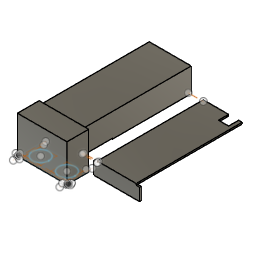
enclosure (Autodesk Fusion 360 design; units mm, degrees)
Autodesk Fusion 360 part; units mm, degrees
sketch "Sketch1" plane through (0, 0, 0) normal (0, 0, 1) x (1, 0, 0)
  line L0 (0, 0) -> (41.5, 0)
  line L1 (41.5, 0) -> (41.5, 105)
  line L2 (41.5, 105) -> (0, 105)
  line L3 (0, 105) -> (0, 0)
  dimension "d1" = 41.5
  dimension "d2" = 105
  constraint horizontal L0
  constraint vertical L1
  constraint horizontal L2
  constraint vertical L3
  constraint coincident L0.start L3.end
  measures "d1" distance of L0.start L0.end
  measures "d2" distance of L0.start L2.end
extrude "Extrude1" add sketch "Sketch1" along normal blind 23 makes body 1
sketch "Sketch2" plane through (0, 0, 0) normal (0, 0, -1) x (1, 0, 0)
  line L0 (0, 0) -> (0, -105)
  line L1 (0, -105) -> (41.5, -105)
  line L2 (41.5, -105) -> (41.5, 0)
  line L3 (41.5, 0) -> (0, 0)
  line L4 (0, -105) -> (41.5, -105)
  line L5 (41.5, -105) -> (41.5, -27)
  line L6 (41.5, -27) -> (0, -27)
  line L7 (0, -27) -> (0, -105)
  dimension "d5" = 78
  constraint horizontal L4
  constraint vertical L5
  constraint horizontal L6
  constraint vertical L7
  constraint coincident L0.end L1.start
  measures "d5" distance of L0.end L6.end
extrude "Extrude2" add sketch "Sketch2" along normal blind 0.75 contours L0 L1 L2 L4 L5 L6 L7 bodies 1
sketch "Sketch3" plane through (0, 0, 0) normal (0, 1, 0) x (1, 0, 0)
  line L0 (-4, 13.7485) -> (45, 13.7485)
  line L1 (45, 13.7485) -> (45, -20.0015)
  line L2 (45, -20.0015) -> (-4, -20.0015)
  line L3 (-4, -20.0015) -> (-4, 13.7485)
  line L4 (20.5, -20.0015) -> (20.5, 1) construction
  dimension "d8" = 49
  dimension "d9" = 33.75
  constraint midpoint L2 L4.start
  constraint perpendicular L2 L4
  constraint symmetric L1 L3 L4
  measures "d8" distance of L0.start L0.end
  measures "d9" distance of L0.start L2.end
extrude "Extrude3" add sketch "Sketch3" against normal blind 21.5 bodies 1
move_face "OffsetFaces1" offset 3 1 faces at (13.6667, -14.3333, 20.0015) on bodies 1
shell "Shell1" thickness 1.5 removed faces 2 at (13.8333, 18, 0) at (13.8333, 79, -0.75) on bodies 1
sketch "Sketch4" plane through (0, 0, -0.75) normal (0, 0, -1) x (1, 0, 0)
  line L0 (40, -103.5) -> (1.5, -103.5)
  line L1 (1.5, -103.5) -> (1.5, -28.5)
  line L2 (1.5, -28.5) -> (40, -28.5)
  line L3 (40, -28.5) -> (40, -103.5)
  line L4 (0, -27) -> (0, -105)
  line L5 (0, -105) -> (41.5, -105)
  line L6 (41.5, -105) -> (41.5, -27)
  line L7 (41.5, -27) -> (0, -27)
surface "Extrude4" add extruded along (0, 1, 0) between 0 and -1.5 1 faces at (27.1667, 28.5, -0.25) separate body on bodies 1 makes body 2
extrude "Extrude5" cut 1 faces at (27.1667, 28, -0.75) along direction (0, 0, 1) blind 1 on bodies 2 bodies 1 2
sketch "Sketch7" plane through (0, 0, 0) normal (0, 1, 0) x (-1, 0, 0)
  line L0 (4, 23.0015) -> (-45, 23.0015)
  line L1 (-45, 23.0015) -> (-45, -13.7485)
  line L2 (-45, -13.7485) -> (4, -13.7485)
  line L3 (4, -13.7485) -> (4, 23.0015)
  line L4 (0, 23) -> (0, 0)
  line L5 (0, 0) -> (-1.5, 0)
  line L6 (-1.5, 0) -> (-40, 0)
  line L7 (-40, 0) -> (-41.5, 0)
  line L8 (-41.5, 0) -> (-41.5, 23)
  line L9 (-41.5, 23) -> (0, 23)
  line L10 (4, -13.7485) -> (2.5, -13.7485) construction
  line L11 (2.5, -13.7485) -> (2.5, -12.2485) construction
  line L12 (-45, -13.7485) -> (-43.5, -13.7485) construction
  line L13 (-43.5, -13.7485) -> (-43.5, -12.2485) construction
  line L14 (4, 0) -> (-45, 0) construction
  dimension "d25" = 1.5
  dimension "d26" = 1.5
  dimension "d27" = 1.5
  dimension "d28" = 1.5
  constraint coincident L2.end L3.start
  constraint perpendicular L3 L10
  constraint perpendicular L10 L11
  constraint coincident L1.end L2.start
  constraint perpendicular L1 L12
  constraint perpendicular L12 L13
  constraint coincident L3 L14.start
  constraint perpendicular L4 L14
  measures "d25" distance of L2.end L10.end
  measures "d26" distance of L10.end L11.end
  measures "d27" distance of L1.end L12.end
  measures "d28" distance of L12.end L13.end
sketch "Sketch13" plane through (0, 0, 0) normal (0, 1, 0) x (-1, 0, 0)
  line L0 (2.5, -12.25) -> (-43.5, -12.25)
  line L1 (-43.5, -12.25) -> (-43.5, 0)
  line L2 (-43.5, 0) -> (2.5, 0)
  line L3 (2.5, 0) -> (2.5, -12.25)
  dimension "d29" = 46
  constraint horizontal L0
  constraint vertical L1
  constraint horizontal L2
  constraint vertical L3
  measures "d29" distance of L0.start L0.end
extrude "Extrude6" cut sketch "Sketch13" against normal blind 2 bodies 1
sketch "Sketch16" plane through (0, 0, -13.7485) normal (0, 0, -1) x (1, 0, 0)
  line L0 (-4, 0) -> (45, 0)
  line L1 (45, 0) -> (45, 21.5)
  line L2 (45, 21.5) -> (-4, 21.5)
  line L3 (-4, 21.5) -> (-4, 0)
  line L4 (-4, 21.5) -> (-2.5, 21.5) construction
  line L5 (45, 21.5) -> (43.5, 21.5) construction
  line L6 (-2.5, 27.1205) -> (-2.5, -5) construction
  line L7 (43.5, 27.0831) -> (43.5, -5) construction
  line L8 (-4, 21.5) -> (-4, 20) construction
  line L9 (45, 21.5) -> (45, 20) construction
  line L10 (-7, 20) -> (47, 20) construction
  line L11 (-2.5, 20) -> (-2.5, 18) construction
  line L12 (-5, 18) -> (46, 18) construction
  line L13 (-2.5, 18) -> (-0.5, 18) construction
  line L14 (-0.5, 22.9727) -> (-0.5, -1) construction
  line L15 (-0.5, 18) -> (15.5, 18) construction
  line L16 (15.5, 18) -> (15.5, 2) construction
  line L17 (15.5, 2) -> (-0.5, 2) construction
  line L18 (-0.5, 2) -> (-0.5, 18) construction
  line L19 (43.5, 20) -> (41.5, 20) construction
  line L20 (41.5, 22.2886) -> (41.5, -1) construction
  line L21 (41.5, 18) -> (25.5, 18) construction
  line L22 (25.5, 18) -> (25.5, 2) construction
  line L23 (25.5, 2) -> (41.5, 2) construction
  line L24 (41.5, 2) -> (41.5, 18) construction
  circle A0 centre (7.5, 10) radius 8
  circle A1 centre (33.5, 10) radius 8
  dimension "d35" = 1.5
  dimension "d36" = 1.5
  dimension "d37" = 2
  dimension "d38" = 16
  dimension "d39" = 16
  dimension "d40" = 2
  dimension "d41" = 16
  dimension "d42" = 16
  dimension "d43" = 8
  dimension "d44" = 8
  constraint coincident L2.end L3.start
  constraint perpendicular L3 L4
  constraint coincident L1.end L2.start
  constraint perpendicular L1 L5
  constraint perpendicular L2 L6
  constraint perpendicular L0 L7
  constraint coincident L3 L8.end
  constraint perpendicular L4 L8
  constraint coincident L1 L9.end
  constraint perpendicular L5 L9
  constraint perpendicular L8 L10
  constraint coincident L10 L11.start
  constraint coincident L6 L11.start
  constraint coincident L6 L11.end
  constraint perpendicular L10 L11
  constraint perpendicular L1 L12
  constraint perpendicular L11 L13
  constraint perpendicular L0 L14
  constraint horizontal L15
  constraint vertical L16
  constraint horizontal L17
  constraint vertical L18
  constraint coincident L10 L19.start
  constraint coincident L7 L19.start
  constraint perpendicular L7 L19
  constraint perpendicular L0 L20
  constraint horizontal L21
  constraint vertical L22
  constraint horizontal L23
  constraint vertical L24
  constraint coincident L20 L21.start
  constraint coincident L12 L21.start
  constraint tangent L17 A0
  constraint tangent L18 A0
  constraint tangent L23 A1
  constraint tangent L22 A1
  measures "d35" distance of L2.end L4.end
  measures "d36" distance of L1.end L5.end
  measures "d37" distance of L11.end L13.end
  measures "d38" distance of L13.end L15.end
  measures "d39" distance of L13.end L17.end
  measures "d40" distance of L19.start L19.end
  measures "d41" distance of L21.start L21.end
  measures "d42" distance of L21.start L23.end
  measures "d43" radius of A0
  measures "d44" radius of A1
extrude "Extrude7" add sketch "Sketch16" against normal blind 2 contours A1 bodies 1
extrude "Extrude8" cut sketch "Sketch16" against normal blind 2 contours A1 bodies 1
extrude "Extrude9" cut sketch "Sketch16" against normal blind 2 contours A0 bodies 1
sketch "Sketch17" plane through (0, 105, 0) normal (0, 1, 0) x (-1, 0, 0)
  line L0 (0, -0.75) -> (0, 23)
  line L1 (0, 23) -> (-41.5, 23)
  line L2 (-41.5, 23) -> (-41.5, -0.75)
  line L3 (-41.5, -0.75) -> (0, -0.75)
  line L4 (-41.5, -0.75) -> (-36.5, -0.75) construction
  line L5 (-36.5, -0.75) -> (-26.5, -0.75)
  line L6 (-26.5, -0.75) -> (-26.5, 4.25)
  line L7 (-26.5, 4.25) -> (-36.5, 4.25)
  line L8 (-36.5, 4.25) -> (-36.5, -0.75)
  dimension "d51" = 5
  dimension "d52" = 10
  dimension "d53" = 5
  constraint coincident L2.end L3.start
  constraint perpendicular L2 L4
  constraint horizontal L5
  constraint vertical L6
  constraint horizontal L7
  constraint vertical L8
  measures "d51" distance of L2.end L4.end
  measures "d52" distance of L4.end L5.end
  measures "d53" distance of L4.end L7.end
extrude "Extrude10" cut sketch "Sketch17" against normal blind 5 contours L3 L5 L6 L7 L8 bodies 1
sketch "Sketch18" plane through (0, 0, 0) normal (0, 0, 1) x (1, 0, 0)
  line L0 (50, 115) -> (88.6, 115)
  line L1 (88.6, 115) -> (88.6, 10)
  line L2 (88.6, 10) -> (50, 10)
  line L3 (50, 10) -> (50, 115)
  dimension "d56" = 38.6
  dimension "d57" = 105
  constraint horizontal L0
  constraint vertical L1
  constraint horizontal L2
  constraint vertical L3
  measures "d56" distance of L0.start L0.end
  measures "d57" distance of L0.start L2.end
extrude "Extrude11" add sketch "Sketch18" against normal blind 1.5 separate body makes body 3
delete_body "RemoveBody1" bodies 2
delete_body "RemoveBody2" bodies 3
sketch "Sketch19" plane through (0, 0, 0) normal (0, 0, 1) x (1, 0, 0)
sketch "Sketch20" plane through (0, 0, 0) normal (0, 0, 1) x (1, 0, 0)
  line L0 (40, 103.5) -> (55, 103.5) construction
  line L1 (40, 0) -> (55, 0) construction
  line L2 (40, -1.5) -> (55, -1.5) construction
  constraint horizontal L0
  constraint horizontal L1
  constraint parallel L1 L2
sketch "Sketch21" plane through (0, 0, 0) normal (0, 0, 1) x (1, 0, 0)
  line L0 (55, 103.5) -> (93.5, 103.5)
  line L1 (93.5, 103.5) -> (93.5, 0)
  line L2 (93.5, 0) -> (55, 0)
  line L3 (55, 0) -> (55, 103.5)
  line L4 (55, 0) -> (51.5, 0) construction
  line L5 (93.5, 0) -> (97, 0) construction
  dimension "d60" = 38.5
  dimension "d61" = 103.5
  dimension "d62" = 3.5
  constraint horizontal L0
  constraint vertical L1
  constraint horizontal L2
  constraint vertical L3
  constraint perpendicular L3 L4
  constraint perpendicular L1 L5
  measures "d60" distance of L0.start L0.end
  measures "d61" distance of L0.start L2.end
  measures "d62" distance of L2.end L4.end
sketch "Sketch24" plane through (0, 0, 0) normal (0, 1, 0) x (1, 0, 0)
  line L0 (51.5, 0) -> (96.9999, 0)
  line L1 (96.9999, 0) -> (96.9999, 12.35)
  line L2 (96.9999, 12.35) -> (51.5, 12.35)
  line L3 (51.5, 12.35) -> (51.5, 0)
  dimension "d63" = 12.35
  constraint horizontal L0
  constraint vertical L1
  constraint horizontal L2
  constraint vertical L3
  measures "d63" distance of L0.start L2.end
extrude "Extrude12" add sketch "Sketch24" against normal blind 1.5 separate body makes body 4
extrude "Extrude13" add sketch "Sketch21" along normal blind 1.5 separate body makes body 5
move_face "OffsetFaces2" offset 1.5 1 faces at (80.6667, 0, 1) on bodies 5
combine "Combine1" operation add target body 4 tool bodies 5
sketch "Sketch25" plane through (0, 0, 0) normal (0, 0, -1) x (1, 0, 0)
  line L0 (93.5, 0) -> (55, 0)
  line L1 (55, 0) -> (55, -103.5)
  line L2 (55, -103.5) -> (93.5, -103.5)
  line L3 (93.5, -103.5) -> (93.5, 0)
  line L4 (93.5, -103.5) -> (90, -103.5) construction
  line L5 (90, -103.5) -> (80, -103.5)
  line L6 (80, -103.5) -> (80, -93.5)
  line L7 (80, -93.5) -> (90, -93.5)
  line L8 (90, -93.5) -> (90, -103.5)
  dimension "d69" = 10
  dimension "d70" = 10
  constraint coincident L2.end L3.start
  constraint coincident L2 L4.end
  constraint perpendicular L3 L4
  constraint horizontal L5
  constraint vertical L6
  constraint horizontal L7
  constraint vertical L8
  measures "d69" distance of L4.end L5.end
  measures "d70" distance of L4.end L7.end
extrude "Extrude14" cut sketch "Sketch25" against normal blind 5 contours L2 L5 L6 L7 L8 bodies 4
named bodies: "enclosure", "bottom-lid"
